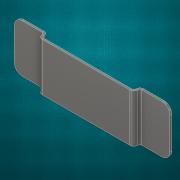
# Autodesk Inventor part: Center Rail Bracket
Saved by Autodesk Inventor 2017 (Build 210142000, 142)
## iProperties
Created: 2017-09-04
Part Number: Center Rail Bracket
Material: Steel, Galvanized
Document SubType Name: Sheet Metal
Designer: Michael
Density: 7.85 g/cm^3
Sheet Metal Rule: Default
Appearance: Galvanized
Author: Michael
Autodesk Inventor part; units mm, degrees
ref_plane "YZ Plane" through (0, 0, 0) normal (1, 0, 0) x (0, 1, 0)
ref_plane "XZ Plane" through (0, 0, 0) normal (0, 1, 0) x (-1, 0, 0)
ref_plane "XY Plane" through (0, 0, 0) normal (0, 0, 1) x (1, 0, 0)
sketch "Sketch1" plane through (0, 0, 0) normal (0, 0, 1) x (1, 0, 0)
  line L0 (-38.1, -19.05) -> (38.1, -19.05)
  line L1 (38.1, -19.05) -> (38.1, 19.05)
  line L2 (38.1, 19.05) -> (-38.1, 19.05)
  line L3 (-38.1, 19.05) -> (-38.1, -19.05)
  line L4 (-38.1, -19.05) -> (38.1, 19.05) construction
  line L5 (38.1, -19.05) -> (-38.1, 19.05) construction
  point P0 (0, 0)
  dimension "d0" = 76.2
  dimension "d1" = 38.1
  measures "d0" distance of L1.end L2.end
  measures "d1" distance of L2.end L0.start
extrude "Plate1" add sketch "Sketch1" along normal blind 1.5875
sketch "Sketch2" plane through (36.5125, -19.05, 1.5875) normal (1, 0, 0) x (0, 1, 0)
  line L0 (38.1, 0) -> (0, 0)
  line L1 (0, 0) -> (0, -4.826)
  line L2 (0, -4.826) -> (38.1, -4.826)
  line L3 (38.1, -4.826) -> (38.1, 0)
  constraints: 6 end point, 1 horizontal, 1 perpendicular, 1 vertical
edge flange "Flange1" height 4.826 angle 90 thickness 1.5875 bend radius 1.5875 thickness toward (1, 0, 0) relief tear relief width 1.5875 relief depth 0.7937 corner gap 1.5875 corner form 0 edges at (38.1, 0, 0) (-38.1, 0, 0) wall of the first edge with corners at (36.5125, 19.05, 1.5875) (36.5125, -19.05, 1.5875) (36.5125, -19.05, -3.2385) (36.5125, 19.05, -3.2385)
bend "Bend1"
corner "Corner1"
sketch "Sketch3" plane through (-38.1, -19.05, -3.2385) normal (0, 0, -1) x (-1, 0, 0)
  line L0 (0, 38.1) -> (0, 0)
  line L1 (0, 0) -> (23.8125, 0)
  line L2 (23.8125, 0) -> (23.8125, 38.1)
  line L3 (23.8125, 38.1) -> (0, 38.1)
  constraints: 6 end point, 1 horizontal, 1 perpendicular, 1 vertical
edge flange "Flange2" height 25.4 angle 90 thickness 1.5875 bend radius 1.5875 thickness toward (0, 0, -1) relief tear relief width 1.5875 relief depth 0.7937 corner gap 1.5875 corner form 0 edges at (-38.1, 0, -3.2385) (38.1, 0, -3.2385) wall of the first edge with corners at (-38.1, 19.05, -3.2385) (-38.1, -19.05, -3.2385) (-61.9125, -19.05, -3.2385) (-61.9125, 19.05, -3.2385)
bend "Bend2"
corner "Corner2"
fillet "Fillet1" radius 6.35 4 edges at (-61.9125, 19.05, -4.0323) (-61.9125, -19.05, -4.0323) (61.9125, -19.05, -4.0323) (61.9125, 19.05, -4.0323)
equation "\"d3\" = BendReliefWidth"
equation "\"d4\" = BendReliefDepth"
equation "\"d5\" = MinimumRemnant"
equation "\"d6\" = BendRadius"
equation "\"d9\" = BendRadius"
equation "\"d10\" = CornerReliefSize"
equation "\"d11\" = GapSize"
equation "\"d12\" = JacobiRadiusSize"
equation "\"d13\" = BendReliefWidth"
equation "\"d14\" = BendReliefDepth"
equation "\"d15\" = MinimumRemnant"
equation "\"d16\" = BendRadius"
equation "\"d19\" = BendRadius"
equation "\"d20\" = CornerReliefSize"
equation "\"d21\" = GapSize"
equation "\"d22\" = JacobiRadiusSize"
equation "\"BendRadius\" = Thickness"
equation "\"BendReliefWidth\" = Thickness"
equation "\"BendReliefDepth\" = 0.5 * Thickness"
equation "\"CornerReliefSize\" = 4 * Thickness"
equation "\"MinimumRemnant\" = 2 * Thickness"
equation "\"TransitionRadius\" = BendRadius"
equation "\"JacobiRadiusSize\" = BendRadius"
equation "\"GapSize\" = Thickness"
equation "\"d2\" = BendRadius"
equation "\"Thickness\" = 1.5875"
body "Solid1"
